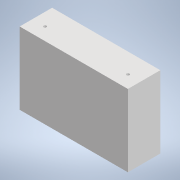
# Autodesk Inventor part: base
Saved by Autodesk Inventor 2022 (Build 260153000, 153)
## iProperties
Created: 2021-06-28
Part Number: base
Material: Generic
Document SubType Name: Sheet Metal
Designer: parag
Density: 1 g/cm^3
Sheet Metal Rule: Default_mm
Appearance: Default
Author: parag
Autodesk Inventor part; units mm, degrees
ref_plane "YZ Plane" through (0, 0, 0) normal (1, 0, 0) x (0, 1, 0)
ref_plane "XZ Plane" through (0, 0, 0) normal (0, 1, 0) x (-1, 0, 0)
ref_plane "XY Plane" through (0, 0, 0) normal (0, 0, 1) x (1, 0, 0)
sketch "Sketch1" plane through (0, 0, 0) normal (0, 0, 1) x (1, 0, 0)
  line L0 (0, 0) -> (300, 0)
  line L1 (300, 0) -> (300, 200)
  line L2 (300, 200) -> (0, 200)
  line L3 (0, 200) -> (0, 0)
  dimension "d0" = 200
  dimension "d1" = 300
  constraints: 8 end point, 2 parallel, 1 horizontal, 1 perpendicular
  measures "d0" distance between parallel lines of L0 L2
  measures "d1" distance between parallel lines of L1 L3
extrude "Extrusion1" add sketch "Sketch1" along normal blind 90
sketch "Sketch2" plane through (0, 0, 0) normal (0, 0, -1) x (-1, 0, 0)
  line L0 (-10, 10) -> (-290, 10)
  line L1 (-290, 10) -> (-290, 190)
  line L2 (-290, 190) -> (-10, 190)
  line L3 (-10, 190) -> (-10, 10)
  line L4 (0, 0) -> (-300, 0) projected
  line L5 (0, 200) -> (0, 0) projected
  dimension "d4" = 180
  dimension "d5" = 280
  dimension "d6" = 10
  dimension "d7" = 10
  constraints: 8 end point, 2 parallel, 1 horizontal, 1 perpendicular
  measures "d4" distance between parallel lines of L2 L0
  measures "d5" distance between parallel lines of L1 L3
  measures "d6" distance between parallel lines of L0 L4
  measures "d7" distance between parallel lines of L3 L5
extrude "Extrusion2" cut sketch "Sketch2" against normal blind 80
sketch "Sketch4" plane through (0, 0, 0) normal (0, 0, -1) x (-1, 0, 0)
  circle A0 centre (-6.4515, 6.4515) radius 1.4515
  circle A1 centre (-6.4515, 193.5485) radius 1.4515
  circle A2 centre (-293.5485, 193.5485) radius 1.4515
  circle A3 centre (-293.5485, 6.4515) radius 1.4515
  line L0 (0, 0) -> (-300, 0) projected
  line L1 (0, 200) -> (0, 0) projected
  line L2 (-300, 200) -> (0, 200) projected
  line L3 (-300, 0) -> (-300, 200) projected
  dimension "d18" = 2.903
  dimension "d19" = 2.903
  dimension "d20" = 2.903
  dimension "d21" = 2.903
  dimension "d22" = 5
  dimension "d23" = 5
  dimension "d24" = 5
  dimension "d25" = 5
  dimension "d26" = 5
  dimension "d27" = 5
  dimension "d28" = 5
  dimension "d29" = 5
  constraints: 4 centre point
  measures "d18" diameter of A0
  measures "d19" diameter of A1
  measures "d20" diameter of A2
  measures "d21" diameter of A3
  measures "d22" distance edge to line of A0 L0
  measures "d23" distance edge to line of A0 L1
  measures "d24" distance edge to line of A1 L1
  measures "d25" distance edge to line of A1 L2
  measures "d26" distance edge to line of A2 L2
  measures "d27" distance edge to line of A2 L3
  measures "d28" distance edge to line of A3 L3
  measures "d29" distance edge to line of A3 L0
extrude "Extrusion4" cut sketch "Sketch4" against normal blind 17 contours A0 | A1 | A2 | A3
sketch "Sketch5" plane through (0, 0, 0) normal (0, -1, 0) x (1, 0, 0)
  circle A0 centre (265, 55) radius 4
  circle A1 centre (35, 55) radius 4
  line L0 (0, 90) -> (300, 90) projected
  line L1 (300, 0) -> (300, 90) projected
  line L2 (0, 0) -> (0, 90) projected
  dimension "d32" = 8
  dimension "d33" = 8
  dimension "d34" = 35
  dimension "d35" = 35
  dimension "d36" = 35
  dimension "d37" = 35
  constraints: 2 centre point
  measures "d32" diameter of A0
  measures "d33" diameter of A1
  measures "d34" distance from line of L0 A0.centre
  measures "d35" distance from line of A0.centre L1
  measures "d36" distance from line of L0 A1.centre
  measures "d37" distance from line of L2 A1.centre
extrude "Extrusion5" cut sketch "Sketch5" against normal through all
sketch "Sketch6" plane through (0, 0, 80) normal (0, 0, -1) x (-1, 0, 0)
  point P0 (0, 0)
sketch "Sketch7" plane through (0, 0, 80) normal (0, 0, -1) x (-1, 0, 0)
  line L0 (-10, 190) -> (-10, 10) projected
  point P0 (0, 0)
sketch "Sketch8" plane through (0, 0, 0) normal (-1, 0, 0) x (0, 0, 1)
  circle A0 centre (45, 100) radius 2.5
  line L0 (0, 0) -> (90, 0) projected
  line L1 (0, 200) -> (0, 0) projected
  dimension "d57" = 5
  dimension "d58" = 100
  dimension "d59" = 45
  constraints: 1 centre point
  measures "d57" diameter of A0
  measures "d58" distance from line of L0 A0.centre
  measures "d59" distance from line of L1 A0.centre
extrude "Extrusion6" cut sketch "Sketch8" against normal blind 10
equation "\"BendRadius\" = Thickness"
equation "\"BendReliefWidth\" = Thickness"
equation "\"BendReliefDepth\" = 0.5 * Thickness"
equation "\"CornerReliefSize\" = 4 * Thickness"
equation "\"MinimumRemnant\" = 2 * Thickness"
equation "\"TransitionRadius\" = BendRadius"
equation "\"JacobiRadiusSize\" = BendRadius"
equation "\"GapSize\" = Thickness"
equation "\"Thickness\" = 0.5"
body "Solid1"
